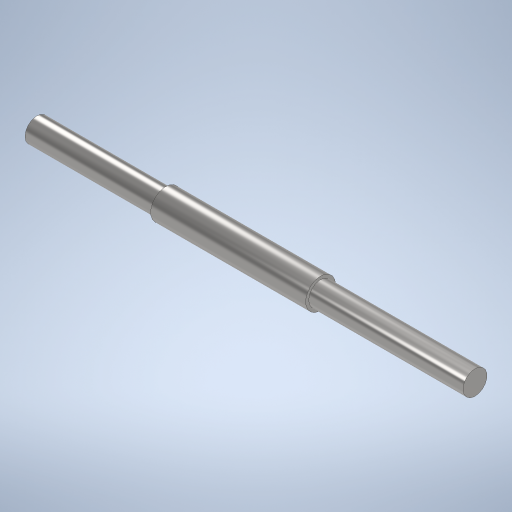
# Autodesk Inventor part: elbow_shaft
Saved by Autodesk Inventor 2024 (Build 280153000, 153)
## iProperties
Created: 2025-08-07
Part Number: elbow_shaft
Material: 鋼、炭素鋼
Document SubType Name: Modeling
Designer: HosodaLab2
Density: 7.85 g/cm^3
Appearance: 半つや出し
Author: HosodaLab2
Autodesk Inventor part; units mm, degrees
ref_plane "YZ Plane" through (0, 0, 0) normal (1, 0, 0) x (0, 1, 0)
ref_plane "XZ Plane" through (0, 0, 0) normal (0, 1, 0) x (-1, 0, 0)
ref_plane "XY Plane" through (0, 0, 0) normal (0, 0, 1) x (1, 0, 0)
sketch "スケッチ1" plane through (0, 0, 0) normal (0, 1, 0) x (-1, 0, 0)
  circle A0 centre (0, 0) radius 5
  dimension "d0" = 10
  constraints: 1 centre point, 1 coincident
  measures "d0" diameter of A0
extrude "押し出し1" add sketch "スケッチ1" along normal blind 51.8
sketch "スケッチ2" plane through (0, 51.8, 0) normal (0, 1, 0) x (1, 0, 0)
  circle A0 centre (0, 0) radius 4
  dimension "d3" = 8
  constraints: 1 centre point, 1 coincident
  measures "d3" diameter of A0
extrude "押し出し2" add sketch "スケッチ2" along normal blind 51.6
sketch "スケッチ3" plane through (0, 0, 0) normal (0, -1, 0) x (1, 0, 0)
  circle A0 centre (0, 0) radius 5 projected
  circle A1 centre (0, 0) radius 4
  dimension "d6" = 8
  constraints: 1 centre point, 1 coincident
  measures "d6" diameter of A1
extrude "押し出し3" add sketch "スケッチ3" along normal blind 43 contours A1
sketch "スケッチ4" plane through (0, 103.4, 0) normal (0, 1, 0) x (1, 0, 0)
  circle A0 centre (0, 0) radius 4 projected
  point P0 (-4, 0)
  constraints: 1 horizontal alignment, 1 other
ref_plane "作業平面1" through (-4, 103.4, 0) normal (-1, 0, 0) x (0, -1, 0)
sketch "スケッチ5" plane through (-4, 103.4, 0) normal (-1, 0, 0) x (0, -1, 0)
  line L0 (5, 1.5) -> (21, 1.5)
  line L1 (21, 1.5) -> (21, -1.5)
  line L2 (21, -1.5) -> (5, -1.5)
  line L3 (5, -1.5) -> (5, 1.5)
  line L4 (5, 1.5) -> (21, -1.5) construction
  line L5 (21, 1.5) -> (5, -1.5) construction
  line L6 (0, 4) -> (0, -4) projected
  point P0 (103.4, 0)
  point P1 (13, 0)
  dimension "d10" = 16
  dimension "d11" = 3
  dimension "d12" = 5
  constraints: 12 end point, 2 midpoint, 2 parallel, 1 horizontal, 1 perpendicular
  measures "d10" distance of L1.end L2.end
  measures "d11" distance of L0.end L1.end
  measures "d12" distance between parallel lines of L6 L3
extrude "押し出し4" cut sketch "スケッチ5" against normal blind 1.8
sketch "スケッチ6" plane through (-4, 103.4, 0) normal (-1, 0, 0) x (0, -1, 0)
  line L0 (125.4, 1.5) -> (141.4, 1.5)
  line L1 (141.4, 1.5) -> (141.4, -1.5)
  line L2 (141.4, -1.5) -> (125.4, -1.5)
  line L3 (125.4, -1.5) -> (125.4, 1.5)
  line L4 (125.4, 1.5) -> (141.4, -1.5) construction
  line L5 (141.4, 1.5) -> (125.4, -1.5) construction
  line L6 (146.4, -4) -> (146.4, 4) projected
  point P0 (103.4, 0)
  point P1 (133.4, 0)
  dimension "d18" = 16
  dimension "d19" = 3
  dimension "d20" = 5
  constraints: 12 end point, 2 midpoint, 2 parallel, 1 horizontal, 1 perpendicular
  measures "d18" distance of L1.end L2.end
  measures "d19" distance of L0.end L1.end
  measures "d20" distance between parallel lines of L6 L1
extrude "押し出し5" cut sketch "スケッチ6" against normal blind 1.8
